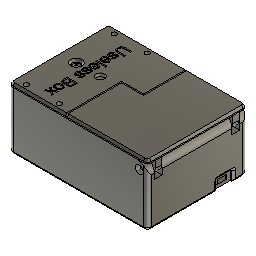
Smart_Useless_Box_box_v1 (Autodesk Fusion 360 design; units mm, degrees)
Autodesk Fusion 360 part; units mm, degrees
(part 1 of 2)
sketch "Base" plane through (0, 0, 0) normal (0, 0, 1) x (1, 0, 0) in component "Box Base"
  line L0 (50, -35) -> (-50, -35)
  line L1 (-50, -35) -> (-50, 35)
  line L2 (-50, 35) -> (50, 35)
  line L3 (50, 35) -> (50, -35)
  line L4 (50, -35) -> (-50, 35) construction
  line L5 (-50, -35) -> (50, 35) construction
  line L6 (50.5, -38.5) -> (-50.5, -38.5)
  line L7 (-53.5, -35.5) -> (-53.5, 35.5)
  line L8 (-50.5, 38.5) -> (50.5, 38.5)
  line L9 (53.5, 35.5) -> (53.5, -35.5)
  line L10 (53.5, -38.5) -> (-53.5, 38.5) construction
  line L11 (-53.5, -38.5) -> (53.5, 38.5) construction
  arc A0 (-53.5, -35.5) -> (-50.5, -38.5) centre (-50.5, -35.5) ccw
  arc A1 (-50.5, 38.5) -> (-53.5, 35.5) centre (-50.5, 35.5) ccw
  arc A2 (53.5, 35.5) -> (50.5, 38.5) centre (50.5, 35.5) ccw
  arc A3 (50.5, -38.5) -> (53.5, -35.5) centre (50.5, -35.5) ccw
  dimension "d5" = 100
  dimension "d6" = 70
  dimension "d7" = 77
  dimension "d8" = 107
  dimension "d9" = 3
  constraint perpendicular L0 L1
  constraint parallel L0 L2
  constraint parallel L1 L3
  constraint horizontal L0
  constraint coincident L4 origin
  constraint coincident L5 origin
  constraint perpendicular L6 L7
  constraint parallel L6 L8
  constraint parallel L7 L9
  constraint horizontal L6
  constraint coincident L10 origin
  constraint coincident L11 origin
  constraint coincident L11.start L6
  constraint coincident L11.start L7
  constraint tangent L6 A0
  constraint tangent L7 A0
  constraint coincident L10.end L7
  constraint coincident L10.end L8
  constraint tangent L7 A1
  constraint tangent L8 A1
  constraint equal A0 A1
  constraint coincident L11.end L8
  constraint coincident L11.end L9
  constraint tangent L8 A2
  constraint tangent L9 A2
  constraint equal A0 A2
  constraint coincident L10.start L9
  constraint coincident L10.start L6
  constraint tangent L9 A3
  constraint tangent L6 A3
  constraint equal A0 A3
  measures "d5" distance of L1.end L2.end
  measures "d6" distance of L0.end L1.end
  measures "d7" distance of L11.start L10.end
  measures "d8" distance of L10.end L11.end
  measures "d9" radius of A0
extrude "Extrude base bottom" add sketch "Base" along normal blind 2.4 contours L0 L1 L2 L3 makes body 1 in component "Box Base"
extrude "Extrude base wall" add sketch "Base" along normal blind 45 bodies 1 in component "Box Base"
chamfer "Chamfer bottom edges" distance 2 angle 35 8 edges at (-52.6213, -37.6213, 0) (-53.5, 0, 0) (-52.6213, 37.6213, 0) (0, 38.5, 0) (52.6213, 37.6213, 0) (53.5, 0, 0) (52.6213, -37.6213, 0) (0, -38.5, 0) measured on face at (-53.4154, -36.2073, 30) measured on face at (-16.8333, -12.8333, 0) measured on face at (-52.3545, 37.8582, 30) measured on face at (-16.8333, -12.8333, 0) measured on face at (51.8747, 38.1665, 30) measured on face at (-16.8333, -12.8333, 0) measured on face at (52, -38.0981, 30) measured on face at (-16.8333, -12.8333, 0) on bodies 1 in component "Box Base"
ref_plane "WorkPlane1" through (-10, 0, 23.7) normal (1, 0, 0) x (0, 1, 0) in component "Box Base"
sketch "Lid mount profile" plane through (-10, 0, 23.7) normal (1, 0, 0) x (0, 1, 0) in component "Box Base"
  line L0 (-35, -21.3) -> (-35, 21.3)
  line L1 (-35, 21.3) -> (35, 21.3)
  line L2 (35, -21.3) -> (35, 21.3)
  line L3 (-29.5, 21.3) -> (-35, 13.4452)
  line L4 (29.5, 21.3) -> (35, 13.4452)
  dimension "d28" = 5.5
  dimension "d29" = 35
  dimension "d30" = 7.8548
  dimension "d31" = 5.5
  dimension "d32" = 35
  constraint coincident L1 L3.start
  constraint coincident L0 L3.end
  constraint coincident L1 L4.start
  constraint coincident L2 L4.end
  measures "d28" distance of L0.end L3.start
  measures "d29" angle of L0 L3
  measures "d30" distance of L0.end L3.end
  measures "d31" distance of L1.end L4.start
  measures "d32" angle of L2 L4
extrude "Extrude lid mount profiles" add sketch "Lid mount profile" against normal up to surface (40 mm away) bodies 1 in component "Box Base"
sketch "Lid mount screws" plane through (0, 0, 45) normal (0, 0, 1) x (-1, 0, 0) in component "Box Base"
  line L0 (10, -35) -> (-50, -35)
  line L1 (-50, -35) -> (-50, 35)
  line L2 (-50, 35) -> (10, 35)
  line L3 (10, 35) -> (10, 29.5)
  line L4 (10, 29.5) -> (50, 29.5)
  line L5 (50, 29.5) -> (50, -29.5)
  line L6 (50, -29.5) -> (10, -29.5)
  line L7 (10, -29.5) -> (10, -35)
  arc A0 (53.5, 35.5) -> (50.5, 38.5) centre (50.5, 35.5) ccw
  line L8 (50.5, 38.5) -> (-50.5, 38.5)
  arc A1 (-50.5, 38.5) -> (-53.5, 35.5) centre (-50.5, 35.5) ccw
  line L9 (-53.5, 35.5) -> (-53.5, -35.5)
  arc A2 (-53.5, -35.5) -> (-50.5, -38.5) centre (-50.5, -35.5) ccw
  line L10 (-50.5, -38.5) -> (50.5, -38.5)
  arc A3 (50.5, -38.5) -> (53.5, -35.5) centre (50.5, -35.5) ccw
  line L11 (53.5, -35.5) -> (53.5, 35.5)
  line L12 (44.5, -29.5) -> (44.5, -38.5) construction
  line L13 (44.5, -34) -> (19, -34) construction
  line L14 (53.5, 0) -> (-53.5, 0) construction
  circle A4 centre (44.5, -34) radius 1.5
  circle A5 centre (19, -34) radius 1.5
  circle A6 centre (19, 34) radius 1.5
  circle A7 centre (44.5, 34) radius 1.5
  dimension "d36" = 9
  dimension "d37" = 9
  dimension "d38" = 3
  dimension "d39" = 3
  constraint coincident L6 L12.start
  constraint coincident L10 L12.end
  constraint perpendicular L10 L12
  constraint midpoint L12 L13.start
  constraint perpendicular L12 L13
  constraint midpoint L11 L14.start
  constraint midpoint L9 L14.end
  constraint coincident L13.start A4.centre
  constraint coincident L13.end A5.centre
  constraint symmetric L14 A4 A7
  constraint symmetric L14 A5 A6
  measures "d36" distance of L11 L12
  measures "d37" distance of L7 L13.end
  measures "d38" diameter of A4
  measures "d39" diameter of A5
extrude "Extrude5" cut sketch "Lid mount screws" against normal blind 15 contours A4 | A5 | A6 | A7 bodies 1 in component "Box Base"
chamfer "Chamfer screw hole edges" distance 1 angle 45 4 edges at (-43.1015, 33.4576, 45) (-17.6015, 33.4576, 45) (-43.1015, -34.5424, 45) (-17.6015, -34.5424, 45) on bodies 1 in component "Box Base"
sketch "Board support" plane through (0, 0, 2.4) normal (0, 0, 1) x (-1, 0, 0) in component "Box Base"
  line L0 (-50, -35) -> (50, -35)
  line L1 (50, -35) -> (50, 35)
  line L2 (50, 35) -> (-50, 35)
  line L3 (-50, 35) -> (-50, -35)
  line L4 (-50, -35) -> (-15, -35)
  line L5 (-15, -35) -> (-15, -8.5)
  line L6 (-15, -8.5) -> (-50, -8.5)
  line L7 (-50, -8.5) -> (-50, -35)
  line L8 (-15, -35) -> (-13, -35)
  line L9 (-13, -6.5) -> (-50, -6.5)
  line L10 (-50, -8.5) -> (-50, -6.5)
  line L11 (-13, -6.5) -> (-13, -35)
  line L12 (-19, -35) -> (-19, -8.5)
  dimension "d50" = 35
  dimension "d51" = 26.5
  dimension "d52" = 2
  dimension "d53" = 2
  dimension "d56" = 4
  constraint horizontal L4
  constraint vertical L5
  constraint horizontal L6
  constraint vertical L7
  constraint coincident L0.start L3.end
  constraint coincident L0 L8.end
  constraint perpendicular L5 L8
  constraint coincident L3 L9.end
  constraint perpendicular L3 L9
  constraint perpendicular L8 L11
  constraint coincident L4 L12.start
  constraint coincident L6 L12.end
  constraint perpendicular L6 L12
  measures "d50" distance of L0.start L4.end
  measures "d51" distance of L0.start L6.end
  measures "d52" distance of L4.end L8.end
  measures "d53" distance of L6 L9
  measures "d56" distance of L5 L12
extrude "Extrude board base support" add sketch "Board support" along normal blind 2 contours L0 L4 L5 L6 L12 bodies 1 in component "Box Base"
extrude "Extrude board wall support" add sketch "Board support" along normal blind 7 contours L0 L3 L5 L6 L8 L9 L10 L11 bodies 1 in component "Box Base"
sketch "USB hole" plane through (53.5, 0, 0) normal (1, 0, 0) x (0, 1, 0) in component "Box Base"
  line L0 (-35.5, 2) -> (35.5, 2)
  line L1 (35.5, 2) -> (35.5, 45)
  line L2 (35.5, 45) -> (-35.5, 45)
  line L3 (-35.5, 45) -> (-35.5, 2)
  line L4 (8.5, 2.4) -> (35, 2.4)
  line L5 (25.5, 2.4) -> (18, 2.4)
  line L6 (18, 2.4) -> (18, 5.6)
  line L7 (18, 5.6) -> (25.5, 5.6)
  line L8 (25.5, 5.6) -> (25.5, 2.4)
  line L9 (25.5, 2.4) -> (18, 5.6) construction
  line L10 (18, 2.4) -> (25.5, 5.6) construction
  line L11 (28, -0.1) -> (15.5, -0.1)
  line L12 (15.5, -0.1) -> (15.5, 7.1)
  line L13 (16.5, 8.1) -> (27, 8.1)
  line L14 (28, 7.1) -> (28, -0.1)
  line L15 (28, -0.1) -> (15.5, 8.1) construction
  line L16 (15.5, -0.1) -> (28, 8.1) construction
  arc A0 (16.5, 8.1) -> (15.5, 7.1) centre (16.5, 7.1) ccw
  arc A1 (28, 7.1) -> (27, 8.1) centre (27, 7.1) ccw
  point P0 (21.75, 4)
  point P1 (21.75, 4)
  dimension "d69" = 7.5
  dimension "d70" = 3.2
  dimension "d71" = 12.5
  dimension "d72" = 8.2
  dimension "d73" = 1
  constraint perpendicular L5 L6
  constraint parallel L5 L7
  constraint parallel L6 L8
  constraint horizontal L5
  constraint coincident L9 P1
  constraint coincident L10 P1
  constraint midpoint L4 L5
  constraint perpendicular L11 L12
  constraint parallel L11 L13
  constraint parallel L12 L14
  constraint horizontal L11
  constraint coincident L15 P1
  constraint coincident L16 P1
  constraint coincident P1 P0
  constraint coincident L15.end L12
  constraint coincident L15.end L13
  constraint tangent L12 A0
  constraint tangent L13 A0
  constraint coincident L16.end L13
  constraint coincident L16.end L14
  constraint tangent L13 A1
  constraint tangent L14 A1
  constraint equal A0 A1
  measures "d69" distance of L6.end L7.end
  measures "d70" distance of L5.end L6.end
  measures "d71" distance of L15.end L16.end
  measures "d72" distance of L11.end L15.end
  measures "d73" radius of A0
extrude "Cut USB hole" cut sketch "USB hole" against normal up to surface (3.5 mm away) contours L4 L5 L6 L7 L8 bodies 1 in component "Box Base"
extrude "Cut USB cable hole" cut sketch "USB hole" against normal blind 2.5 contours L0 L4 L5 L12 L14 | L0 L11 L12 L14 | L4 L6 L7 L8 L12 L13 L14 A0 A1 bodies 1 in component "Box Base"
chamfer "Chamfer USB edges" distance 2 angle 35 5 edges at (53.5, 15.5, 4.55) (53.5, 15.7929, 7.8071) (53.5, 21.75, 8.1) (53.5, 27.7071, 7.8071) (53.5, 28, 4.55) measured on face at (53.5, 5.3487, 32.6637) measured on face at (53.5, 5.3487, 32.6637) measured on face at (53.5, 5.3487, 32.6637) measured on face at (53.5, 5.3487, 32.6637) measured on face at (53.5, 5.3487, 32.6637) on bodies 1 in component "Box Base"
sketch "Shaft" plane through (0, -38.5, 0) normal (0, -1, 0) x (1, 0, 0) in component "Box Base"
  line L0 (-50.5, 2) -> (50.5, 2)
  line L1 (50.5, 2) -> (50.5, 45)
  line L2 (50.5, 45) -> (-50.5, 45)
  line L3 (-50.5, 45) -> (-50.5, 2)
  line L4 (53.5, 7.1) -> (53.5, 2)
  line L5 (53.5, 2) -> (53.5, 45)
  line L6 (53.5, 45) -> (53.5, 2)
  line L7 (53.5, 2) -> (53.5, 7.1)
  line L8 (53.5, 7.1) -> (53.5, 10.1)
  line L9 (53.5, 7.1) -> (53.5, 10.1)
  line L10 (-10, 45) -> (50, 45)
  line L11 (50, 2.4) -> (50, 45)
  circle A0 centre (47.3, 38.8) radius 1.5
  circle A1 centre (47.3, 38.8) radius 3.2
  circle A2 centre (47.3, 38.8) radius 6.2
  line L12 (41.1, 38.8) -> (41.1, 45)
  line L13 (42.2213, 35.2438) -> (50, 24.1346)
  spline S0 degree 5 poles (45.3, 45) (45.5877, 44.9597) (46.1522, 44.8682) (46.9666, 44.6986) (47.9866, 44.4066) (49.1443, 43.9243) (50.1744, 43.3144) (51.0663, 42.5663) (51.8144, 41.6744) (52.4243, 40.6443) (52.9066, 39.4866) (53.1986, 38.4666) (53.3682, 37.6522) (53.4597, 37.0877) (53.5, 36.8) knots 0 0 0 0 0 0 0.1 0.2 0.3 0.4 0.5 0.6 0.7 0.8 0.9 1 1 1 1 1 1
  line L14 (47.3, 38.8) -> (53.5, 45) construction
  line L15 (53.5, 45) -> (50, 45)
  point P0 (51.0304, 42.5304)
  dimension "d99" = 3
  dimension "d100" = 6.4
  dimension "d101" = 12.4
  dimension "d103" = 6.2
  dimension "d104" = 6.2
  dimension "d105" = 35
  dimension "d123" = 8.2
  dimension "d124" = 8.2
  constraint concentric A0 A1
  constraint concentric A0 A2
  constraint coincident A2 L12.start
  constraint tangent A2 L12
  constraint coincident L10 L12.end
  constraint perpendicular L2 L12
  constraint coincident A2 L13.start
  constraint tangent A2 L13
  constraint coincident L11 L13.end
  constraint coincident L10 S0.start
  constraint coincident L5 S0.end
  constraint coincident A0.centre A1.centre
  constraint coincident L5.end L6.start
  constraint coincident P0 L14
  constraint coincident L10.end L11.end
  measures "d99" diameter of A0
  measures "d100" diameter of A1
  measures "d101" diameter of A2
  measures "d103" distance of L2 A0.centre
  measures "d104" distance of L6 A0.centre
  measures "d105" angle of L11 L13
  measures "d123" distance of S0.start L5.end
  measures "d124" distance of S0.end L5.end
extrude "Extrude20" cut sketch "Shaft" against normal up to surface (77 mm away) contours L1 A2 S0 | L5 L6 A2 S0 | L1 L11 A2 S0 | L1 L5 L6 A2 L15 | L2 L10 A2 S0 | L1 L2 L11 A2 L15 | L11 A2 S0 | L2 L10 L11 A2 picked at (52.3629, 41.2358) bodies 1 in component "Box Base"
extrude "Extrude shaft case" add sketch "Shaft" against normal up to surface (73.5 mm away) contours L11 A1 A2 S0 | L11 A2 L13 | L2 L10 A2 L12 S0 | L11 A1 | L2 L10 A2 S0 | L11 A2 S0 | L2 L10 L11 A2 | A0 picked at (49.6, 38.8) bodies 1 in component "Box Base"
extrude "Cut shaft screw hole" cut sketch "Shaft" against normal up to surface (77 mm away) contours A0 bodies 1 in component "Box Base"
extrude "Cut shaft screw head hole front" cut sketch "Shaft" against normal blind 3.5 contours L11 A1 | L11 A1 bodies 1 in component "Box Base"
sketch "Shaft head hole back" plane through (0, 38.5, 0) normal (0, 1, 0) x (-1, 0, 0) in component "Box Base"
  circle A0 centre (-47.3, 38.8) radius 1.5
  line L0 (-50.5, 2) -> (50.5, 2)
  line L1 (50.5, 2) -> (50.5, 45)
  line L2 (50.5, 45) -> (-45.3, 45)
  line L3 (-50.5, 43.0074) -> (-50.5, 2)
  circle A1 centre (-47.3, 38.8) radius 3.2
  spline S0 degree 5 poles (-45.3, 45) (-45.5877, 44.9597) (-46.1522, 44.8682) (-46.9666, 44.6986) (-47.9866, 44.4066) (-49.0021, 43.9836) (-49.7129, 43.5838) (-50.175, 43.2634) (-50.43, 43.0639) (-50.5, 43.0074) knots 0 0 0 0 0 0 0.1 0.2 0.3 0.4 0.438574 0.438574 0.438574 0.438574 0.438574 0.438574
extrude "Cut shaft screw head hole back" cut sketch "Shaft head hole back" against normal blind 3.5 contours A1 bodies 1 in component "Box Base"
sketch "Shaft top mount holes" plane through (0, 0, 45) normal (0, 0, 1) x (-1, 0, 0) in component "Box Base"
  line L0 (50.5, 38.5) -> (-50, 38.5)
  line L1 (-45.3, -38.5) -> (50.5, -38.5)
  arc A0 (50.5, -38.5) -> (53.5, -35.5) centre (50.5, -35.5) ccw
  line L2 (53.5, -35.5) -> (53.5, 35.5)
  arc A1 (53.5, 35.5) -> (50.5, 38.5) centre (50.5, 35.5) ccw
  line L3 (-41.1, 35) -> (10, 35)
  line L4 (10, 35) -> (10, 29.5)
  line L5 (10, 29.5) -> (50, 29.5)
  line L6 (50, 29.5) -> (50, -29.5)
  line L7 (50, -29.5) -> (10, -29.5)
  line L8 (10, -29.5) -> (10, -35)
  line L9 (10, -35) -> (-41.1, -35)
  line L10 (-41.1, -35) -> (-41.1, 35)
  circle A2 centre (44.5, 34) radius 2.5
  circle A3 centre (44.5, -34) radius 2.5
  circle A4 centre (19, -34) radius 2.5
  circle A5 centre (19, 34) radius 2.5
  line L11 (-41.1, -33) -> (-53.5, -33)
  line L12 (-53.5, -33) -> (-53.5, -27)
  line L13 (-53.5, -27) -> (-41.1, -27)
  line L14 (-41.1, -27) -> (-41.1, -33)
  line L15 (-45.3, -35) -> (-45.3, -38.5)
  line L16 (-50, 38.5) -> (-50, -35)
  line L17 (-50, -35) -> (-45.3, -35)
  line L18 (53.5, 0) -> (-50, 0) construction
  line L19 (-41.1, 33) -> (-53.5, 33)
  line L20 (-53.5, 33) -> (-53.5, 27)
  line L21 (-53.5, 27) -> (-41.1, 27)
  line L22 (-41.1, 27) -> (-41.1, 33)
  dimension "d115" = 6
  dimension "d130" = 2
  constraint horizontal L11
  constraint vertical L12
  constraint horizontal L13
  constraint vertical L14
  constraint midpoint L2 L18.start
  constraint coincident L16 L18.end
  constraint perpendicular L16 L18
  constraint symmetric L11.start L18 L19.start
  constraint symmetric L11.end L18 L19.end
  constraint symmetric L12.end L18 L20.end
  constraint symmetric L13.end L18 L21.end
  measures "d115" distance of L11 L13
  measures "d130" distance of L11 L15.start
extrude "Cut shaft top mount holes" cut sketch "Shaft top mount holes" against normal blind 12.4 contours L10 L16 L19 L21 L22 | L16 L19 L20 L21 | L11 L12 L13 L16 | L10 L11 L13 L14 L16 bodies 1 in component "Box Base"
extrude "Cut shaft roundover" cut sketch "Shaft" against normal up to surface (77 mm away) contours L1 A2 S0 | L5 L6 A2 S0 | L1 L11 A2 S0 | L1 L5 L6 A2 L15 | L2 L10 A2 S0 | L1 L2 L11 A2 L15 | L11 A2 S0 | L2 L10 L11 A2 picked at (52.3629, 41.2358) bodies 1 in component "Box Base"
sketch "Top" plane through (0, 0, 45) normal (0, 0, 1) x (-1, 0, 0) in component "Fixed Lid"
  circle A0 centre (44.5, 34) radius 2.5
  circle A1 centre (44.5, -34) radius 2.5
  circle A2 centre (19, -34) radius 2.5
  circle A3 centre (19, 34) radius 2.5
  line L0 (-45.3, 38.5) -> (-45.3, 33)
  line L1 (-45.3, 33) -> (-41.1, 33)
  line L2 (-41.1, 33) -> (-41.1, 35)
  line L3 (-41.1, 35) -> (10, 35)
  line L4 (10, 35) -> (10, 29.5)
  line L5 (10, 29.5) -> (50, 29.5)
  line L6 (50, 29.5) -> (50, -29.5)
  line L7 (50, -29.5) -> (10, -29.5)
  line L8 (10, -29.5) -> (10, -35)
  line L9 (10, -35) -> (-41.1, -35)
  line L10 (-41.1, -35) -> (-41.1, -33)
  line L11 (-41.1, -33) -> (-45.3, -33)
  line L12 (-45.3, -33) -> (-45.3, -38.5)
  line L13 (-45.3, -38.5) -> (50.5, -38.5)
  arc A4 (50.5, -38.5) -> (53.5, -35.5) centre (50.5, -35.5) ccw
  line L14 (53.5, -35.5) -> (53.5, 35.5)
  arc A5 (53.5, 35.5) -> (50.5, 38.5) centre (50.5, 35.5) ccw
  line L15 (50.5, 38.5) -> (-45.3, 38.5)
  line L16 (10, -38.5) -> (10, 38.5)
  circle A6 centre (19, -34) radius 1.9
  circle A7 centre (44.5, -34) radius 1.9
  circle A8 centre (44.5, 34) radius 1.9
  circle A9 centre (19, 34) radius 1.9
  line L17 (0, 0) -> (53.5, 0) construction
  circle A10 centre (21.5, 0) radius 3.35
  line L18 (-7, -38.5) -> (-7, -5)
  line L19 (-7, -5) -> (10, -5)
  circle A11 centre (40, 0) radius 3.1
  line L20 (48, -5) -> (32, -5)
  line L21 (32, -5) -> (32, 16)
  line L22 (32, 16) -> (48, 16)
  line L23 (48, 16) -> (48, -5)
  line L24 (50, 18) -> (50, -7)
  line L25 (50, -7) -> (30, -7)
  line L26 (30, -7) -> (30, 18)
  line L27 (30, 18) -> (50, 18)
  line L28 (50, -29.5) -> (50, 29.5) construction
  line L29 (40, -5) -> (40, 16) construction
  dimension "d132" = 3.8
  dimension "d133" = 3.8
  dimension "d134" = 3.8
  dimension "d135" = 3.8
  dimension "d138" = 6.7
  dimension "d140" = 11.5
  dimension "d143" = 17
  dimension "d145" = 5
  dimension "d152" = 6.2
  dimension "d156" = 16
  dimension "d157" = 21
  dimension "d160" = 5
  constraint coincident L13 L16.start
  constraint coincident L15 L16.end
  constraint perpendicular L15 L16
  constraint collinear L8 L16
  constraint concentric A2 A6
  constraint concentric A1 A7
  constraint concentric A0 A8
  constraint concentric A3 A9
  constraint coincident L17.start origin
  constraint midpoint L14 L17.end
  constraint coincident L17 A10.centre
  constraint coincident L13 L18.start
  constraint perpendicular L13 L18
  constraint coincident L16 L19.end
  constraint perpendicular L16 L19
  constraint coincident L17 A11.centre
  constraint horizontal L20
  constraint vertical L21
  constraint horizontal L22
  constraint vertical L23
  constraint coincident L6.end L7.start
  constraint coincident L5.end L6.start
  constraint coincident L24 L5.end
  constraint midpoint L20 L29.start
  constraint midpoint L22 L29.end
  constraint coincident A11.centre L29
  measures "d132" diameter of A6
  measures "d133" diameter of A7
  measures "d134" diameter of A8
  measures "d135" diameter of A9
  measures "d138" diameter of A10
  measures "d140" distance of L16 A10.centre
  measures "d143" distance of L16 L18
  measures "d145" distance of L17.start L19
  measures "d152" diameter of A11
  measures "d156" distance of L20.start L20.end
  measures "d157" distance of L20.start L22.end
  measures "d160" distance of A11.centre L20
extrude "Extrude fixed lid" add sketch "Top" along normal blind 2.6 separate body contours A0 | A1 | A2 | A3 | L4 L5 L6 L7 L8 L13 A4 L14 A5 L15 L16 L24 | L5 L6 L7 L16 L25 L26 L27 | L8 L9 L16 L18 L19 | L6 L24 L25 L26 L27 | L9 L13 L16 L18 | L20 L21 L22 L23 makes body 2 in component "Fixed Lid"
chamfer "Chamfer1" distance 1.2 angle 55 6 edges at (-21.75, 38.5, 47.6) (-52.6213, 37.6213, 47.6) (-53.5, 0, 47.6) (-52.6213, -37.6213, 47.6) (-30.25, -38.5, 47.6) (-37.1098, -1.121, 47.6) measured on face at (-6.8691, 24.2359, 47.6) measured on face at (-6.8691, 24.2359, 47.6) measured on face at (-6.8691, 24.2359, 47.6) measured on face at (-6.8691, 24.2359, 47.6) measured on face at (-6.8691, 24.2359, 47.6) measured on face at (-6.8691, 24.2359, 47.6) on bodies 2 in component "Fixed Lid"
sketch "Bottom" plane through (0, 0, 45) normal (0, 0, -1) x (1, 0, 0) in component "Fixed Lid"
  circle A0 centre (-21.5, 0) radius 3.35
  circle A1 centre (-40, 0) radius 3.1
  circle A2 centre (-19, 34) radius 1.9
  circle A3 centre (-44.5, 34) radius 1.9
  circle A4 centre (-44.5, -34) radius 1.9
  circle A5 centre (-19, -34) radius 1.9
  line L0 (-50.5, -38.5) -> (7, -38.5)
  line L1 (7, -38.5) -> (7, -5)
  line L2 (7, -5) -> (-10, -5)
  line L3 (-10, -5) -> (-10, 38.5)
  line L4 (-10, 38.5) -> (-50.5, 38.5)
  arc A6 (-50.5, 38.5) -> (-53.5, 35.5) centre (-50.5, 35.5) ccw
  line L5 (-53.5, 35.5) -> (-53.5, -35.5)
  arc A7 (-53.5, -35.5) -> (-50.5, -38.5) centre (-50.5, -35.5) ccw
  line L6 (-50, -7) -> (-30, -7)
  line L7 (-30, -7) -> (-30, 18)
  line L8 (-50, 18) -> (-50, -7)
  line L9 (-30, 18) -> (-50, 18)
  line L10 (-48, -5) -> (-32, -5)
  line L11 (-32, -5) -> (-32, 16)
  line L12 (-48, 16) -> (-48, -5)
  line L13 (-32, 16) -> (-48, 16)
  line L14 (7, -38.5) -> (7, -5)
  line L15 (7, -23.5) -> (1.6, -23.5)
  line L16 (1.6, -23.5) -> (1.6, -15)
  line L17 (1.6, -15) -> (7, -15)
  line L18 (7, -15) -> (7, -23.5)
  line L19 (-21.6, -23.5) -> (-27, -23.5)
  line L20 (-27, -23.5) -> (-27, -15)
  line L21 (-27, -15) -> (-21.6, -15)
  line L22 (-21.6, -15) -> (-21.6, -23.5)
  line L23 (-42.6, -5) -> (-48, -5)
  line L24 (-48, -5) -> (-48, 0.4)
  line L25 (-48, 0.4) -> (-42.6, 0.4)
  line L26 (-42.6, 0.4) -> (-42.6, -5)
  line L27 (-42.6, -5) -> (-48, 0.4) construction
  line L28 (-48, -5) -> (-42.6, 0.4) construction
  line L29 (-32, -5) -> (-37.4, -5)
  line L30 (-37.4, -5) -> (-37.4, 0.4)
  line L31 (-37.4, 0.4) -> (-32, 0.4)
  line L32 (-32, 0.4) -> (-32, -5)
  line L33 (-32, -5) -> (-37.4, 0.4) construction
  line L34 (-37.4, -5) -> (-32, 0.4) construction
  circle A8 centre (-45.3, -2.3) radius 1.25
  circle A9 centre (-34.7, -2.3) radius 1.25
  arc A10 (-42.6, -2.3) -> (-45.3, 0.4) centre (-45.3, -2.3) ccw
  arc A11 (-34.7, 0.4) -> (-37.4, -2.3) centre (-34.7, -2.3) ccw
  point P0 (-45.3, -2.3)
  point P1 (-34.7, -2.3)
  dimension "d170" = 15
  dimension "d171" = 8.5
  dimension "d172" = 5.4
  dimension "d173" = 15
  dimension "d174" = 8.5
  dimension "d175" = 5.4
  dimension "d176" = 23.2
  dimension "d192" = 5.4
  dimension "d193" = 5.4
  dimension "d194" = 5.4
  dimension "d195" = 5.4
  dimension "d196" = 2.5
  dimension "d197" = 2.5
  constraint horizontal L15
  constraint vertical L16
  constraint horizontal L17
  constraint vertical L18
  constraint coincident L14 L15.start
  constraint horizontal L19
  constraint vertical L20
  constraint horizontal L21
  constraint vertical L22
  constraint perpendicular L23 L24
  constraint parallel L23 L25
  constraint parallel L24 L26
  constraint horizontal L23
  constraint coincident L27 P0
  constraint coincident L28 P0
  constraint coincident L10.start L12.end
  constraint perpendicular L29 L30
  constraint parallel L29 L31
  constraint parallel L30 L32
  constraint horizontal L29
  constraint coincident L33 P1
  constraint coincident L34 P1
  constraint coincident L10.end L11.start
  constraint coincident P0 A8.centre
  constraint coincident P1 A9.centre
  constraint midpoint L26 A10.start
  constraint midpoint L25 A10.end
  constraint midpoint L30 A11.end
  constraint midpoint L31 A11.start
  measures "d170" distance of origin L17
  measures "d171" distance of L15.end L16.end
  measures "d172" distance of L15.start L15.end
  measures "d173" distance of origin L21
  measures "d174" distance of L19.end L20.end
  measures "d175" distance of L19.start L19.end
  measures "d176" distance of L16 L22
  measures "d192" distance of L24.end L25.end
  measures "d193" distance of L10.start L24.end
  measures "d194" distance of L30.end L31.end
  measures "d195" distance of L29.end L30.end
  measures "d196" diameter of A8
  measures "d197" diameter of A9
extrude "Extrude6" add sketch "Bottom" along normal blind 1.6 contours A1 L10 L11 L29 L30 L31 L32 A11 | A1 A11 | A1 A10 | A1 L10 L12 L23 L24 L25 L26 A10 bodies 2 in component "Fixed Lid"
extrude "Extrude motor mounts" add sketch "Bottom" along normal blind 13 contours L1 L14 L15 L16 L17 L18 | L19 L20 L21 L22 bodies 2 in component "Fixed Lid"
extrude "Extrude sensor wall support" add sketch "Bottom" along normal blind 4 contours L6 L7 L8 L9 bodies 2 in component "Fixed Lid"
sketch "Motor mounts" plane through (0, 15, 0) normal (0, -1, 0) x (1, 0, 0) in component "Fixed Lid"
  line L0 (7, 45) -> (1.6, 45)
  line L1 (1.6, 45) -> (1.6, 32)
  line L2 (1.6, 32) -> (7, 32)
  line L3 (7, 32) -> (7, 45)
  line L4 (-21.6, 45) -> (-27, 45)
  line L5 (-27, 45) -> (-27, 32)
  line L6 (-27, 32) -> (-21.6, 32)
  line L7 (-21.6, 32) -> (-21.6, 45)
  line L8 (-24.3, 45) -> (-24.3, 32) construction
  line L9 (4.3, 45) -> (4.3, 32) construction
  circle A0 centre (-24.3, 38.7) radius 1.1
  circle A1 centre (4.3, 38.7) radius 1.1
  line L10 (-27, 45) -> (-21.6, 45)
  line L11 (1.6, 45) -> (7, 45)
  dimension "d179" = 2.2
  dimension "d180" = 2.2
  dimension "d182" = 6.3
  dimension "d183" = 6.3
  constraint midpoint L4 L8.start
  constraint midpoint L6 L8.end
  constraint midpoint L0 L9.start
  constraint midpoint L2 L9.end
  constraint coincident L8 A0.centre
  constraint coincident L9 A1.centre
  measures "d179" diameter of A0
  measures "d180" diameter of A1
  measures "d182" distance of A0.centre L10
  measures "d183" distance of A1.centre L11
extrude "Cut motor mount holes" cut sketch "Motor mounts" against normal up to surface (8.5 mm away) contours A0 | A1 bodies 2 in component "Fixed Lid"
fillet "Fillet1" radius 4 3 edges at (-27, 19.25, 45) (-24.3, 23.5, 45) (4.3, 23.5, 45) on bodies 2 in component "Fixed Lid"
sketch "Text" plane through (0, 0, 47.6) normal (0, 0, 1) x (-1, 0, 0) in component "Fixed Lid"
  circle A0 centre (21.5, 0) radius 3.35
  circle A1 centre (19, 34) radius 1.9
  circle A2 centre (44.5, 34) radius 1.9
  circle A3 centre (44.5, -34) radius 1.9
  circle A4 centre (19, -34) radius 1.9
  line L0 (-7, -37.3) -> (50.5, -37.3)
  arc A5 (50.5, -37.3) -> (52.3, -35.5) centre (50.5, -35.5) ccw
  line L1 (52.3, -35.5) -> (52.3, 35.5)
  arc A6 (52.3, 35.5) -> (50.5, 37.3) centre (50.5, 35.5) ccw
  line L2 (50.5, 37.3) -> (10, 37.3)
  line L3 (10, 37.3) -> (10, -5)
  line L4 (10, -5) -> (-7, -5)
  line L5 (-7, -5) -> (-7, -37.3)
  circle A7 centre (40, 0) radius 4.3
  line L6 (33.8228, -28.9087) -> (33.8228, 31.2798) construction
  line L7 (33.8228, 31.2798) -> (22.8228, 31.2798) construction
  line L8 (22.8228, 31.2798) -> (22.8228, -28.9087) construction
  line L9 (22.8228, -28.9087) -> (33.8228, -28.9087) construction
  text T0 "Useless Box" font "Arial" height 11 align ink ink in box 0 x 0 at (33.8228, -28.9087) x (0, 1) y (-1, 0) spacing 1 height is em
  constraint perpendicular L6 L7
  constraint parallel L6 L8
  constraint parallel L7 L9
extrude "Extrude5'" cut sketch "Text" against normal blind 1 text T0 bodies 2 in component "Fixed Lid"
sketch "Bottom (2)" plane through (0, 0, 45) normal (0, 0, 1) x (-1, 0, 0) in component "Moving Lid"
  circle A0 centre (44.5, 34) radius 2.5
  circle A1 centre (44.5, -34) radius 2.5
  circle A2 centre (19, -34) radius 2.5
  circle A3 centre (19, 34) radius 2.5
  line L0 (-45.3, 38.5) -> (-45.3, 33)
  line L1 (-45.3, 33) -> (-41.1, 33)
  line L2 (-41.1, 33) -> (-41.1, 35)
  line L3 (-41.1, 35) -> (10, 35)
  line L4 (10, 35) -> (10, 29.5)
  line L5 (10, 29.5) -> (50, 29.5)
  line L6 (50, 29.5) -> (50, -29.5)
  line L7 (50, -29.5) -> (10, -29.5)
  line L8 (10, -29.5) -> (10, -35)
  line L9 (10, -35) -> (-41.1, -35)
  line L10 (-41.1, -35) -> (-41.1, -33)
  line L11 (-41.1, -33) -> (-45.3, -33)
  line L12 (-45.3, -33) -> (-45.3, -38.5)
  line L13 (-45.3, -38.5) -> (50.5, -38.5)
  arc A4 (50.5, -38.5) -> (53.5, -35.5) centre (50.5, -35.5) ccw
  line L14 (53.5, -35.5) -> (53.5, 35.5)
  arc A5 (53.5, 35.5) -> (50.5, 38.5) centre (50.5, 35.5) ccw
  line L15 (50.5, 38.5) -> (-45.3, 38.5)
  circle A6 centre (40, 0) radius 4.3
  line L16 (-7, -37.3) -> (50.5, -37.3)
  arc A7 (50.5, -37.3) -> (52.3, -35.5) centre (50.5, -35.5) ccw
  line L17 (52.3, -35.5) -> (52.3, 35.5)
  arc A8 (52.3, 35.5) -> (50.5, 37.3) centre (50.5, 35.5) ccw
  line L18 (50.5, 37.3) -> (10, 37.3)
  line L19 (10, 37.3) -> (10, -5)
  line L20 (10, -5) -> (-7, -5)
  line L21 (-7, -5) -> (-7, -37.3)
  circle A9 centre (19, 34) radius 1.9
  circle A10 centre (44.5, -34) radius 1.9
  circle A11 centre (19, -34) radius 1.9
  circle A12 centre (21.5, 0) radius 3.35
  circle A13 centre (44.5, 34) radius 1.9
  spline S0 degree 3 poles (32.3472, -24.2366) (32.0988, -24.0953) (31.4834, -23.7453) (30.7695, -23.7469) (30.3438, -23.7478) knots 0 0 0 0 0.084501 0.209307 0.209307 0.209307 0.209307
  line L22 (30.3438, -23.7478) -> (25.7998, -23.7478)
  line L23 (25.7998, -23.7478) -> (25.7998, -22.7058)
  line L24 (25.7998, -22.7058) -> (30.3492, -22.7058)
  spline S1 degree 3 poles (30.3492, -22.7058) (30.7068, -22.7108) (31.3475, -22.7197) (31.9626, -22.8963) (32.2344, -22.9744) knots 0 0 0 0 0.106693 0.191173 0.191173 0.191173 0.191173
  spline S2 degree 3 poles (32.2344, -22.9744) (32.4581, -23.0849) (32.918, -23.3121) (33.2169, -23.7295) (33.3704, -23.9439) knots 0 0 0 0 0.073668 0.151407 0.151407 0.151407 0.151407
  spline S3 degree 3 poles (33.3704, -23.9439) (33.4978, -24.2095) (33.7761, -24.7895) (33.7969, -25.4341) (33.8081, -25.7835) knots 0 0 0 0 0.087434 0.190938 0.190938 0.190938 0.190938
  spline S4 degree 3 poles (33.8081, -25.7835) (33.7983, -26.1236) (33.7802, -26.7511) (33.5378, -27.3289) (33.4268, -27.5935) knots 0 0 0 0 0.101025 0.186391 0.186391 0.186391 0.186391
  spline S5 degree 3 poles (33.4268, -27.5935) (33.2862, -27.811) (33.0068, -28.2432) (32.55, -28.4802) (32.323, -28.5979) knots 0 0 0 0 0.076238 0.151547 0.151547 0.151547 0.151547
  spline S6 degree 3 poles (32.323, -28.5979) (32.0401, -28.6853) (31.3983, -28.8837) (30.7255, -28.8933) (30.3492, -28.8987) knots 0 0 0 0 0.088394 0.200567 0.200567 0.200567 0.200567
  line L25 (30.3492, -28.8987) -> (25.7998, -28.8987)
  line L26 (25.7998, -28.8987) -> (25.7998, -27.8567)
  line L27 (25.7998, -27.8567) -> (30.3438, -27.8567)
  spline S7 degree 3 poles (30.3438, -27.8567) (30.6429, -27.8556) (31.1555, -27.8538) (31.6498, -27.7213) (31.8558, -27.666) knots 0 0 0 0 0.08922 0.152949 0.152949 0.152949 0.152949
  spline S8 degree 3 poles (31.8558, -27.666) (32.0088, -27.5906) (32.3166, -27.4388) (32.5085, -27.154) (32.605, -27.0108) knots 0 0 0 0 0.050236 0.10109 0.10109 0.10109 0.10109
  spline S9 degree 3 poles (32.605, -27.0108) (32.6817, -26.8413) (32.8449, -26.4807) (32.8601, -26.0847) (32.8682, -25.8748) knots 0 0 0 0 0.055274 0.117592 0.117592 0.117592 0.117592
  spline S10 degree 3 poles (32.8682, -25.8748) (32.8605, -25.5342) (32.847, -24.9324) (32.4985, -24.4472) (32.3472, -24.2366) knots 0 0 0 0 0.099283 0.175461 0.175461 0.175461 0.175461
  spline S11 degree 3 poles (33.0079, -13.1936) (32.9979, -13.0252) (32.9786, -12.6994) (32.81, -12.4206) (32.7286, -12.2859) knots 0 0 0 0 0.049772 0.096252 0.096252 0.096252 0.096252
  spline S12 degree 3 poles (32.7286, -12.2859) (32.6139, -12.1645) (32.3629, -11.8985) (32.0221, -11.7632) (31.837, -11.6897) knots 0 0 0 0 0.049501 0.108413 0.108413 0.108413 0.108413
  line L28 (31.837, -11.6897) -> (31.9605, -10.6907)
  spline S13 degree 3 poles (31.9605, -10.6907) (32.2331, -10.7825) (32.7605, -10.9601) (33.1373, -11.3687) (33.3194, -11.5662) knots 0 0 0 0 0.084738 0.163983 0.163983 0.163983 0.163983
  spline S14 degree 3 poles (33.3194, -11.5662) (33.4602, -11.8026) (33.7593, -12.3046) (33.7877, -12.8896) (33.8028, -13.199) knots 0 0 0 0 0.081309 0.172615 0.172615 0.172615 0.172615
  spline S15 degree 3 poles (33.8028, -13.199) (33.777, -13.5883) (33.7276, -14.3328) (33.2567, -14.9088) (33.032, -15.1836) knots 0 0 0 0 0.113831 0.217681 0.217681 0.217681 0.217681
  spline S16 degree 3 poles (33.032, -15.1836) (32.7342, -15.3971) (32.0906, -15.8584) (31.2966, -15.8964) (30.8702, -15.9168) knots 0 0 0 0 0.107682 0.232636 0.232636 0.232636 0.232636
  spline S17 degree 3 poles (30.8702, -15.9168) (30.4295, -15.8967) (29.6116, -15.8593) (28.9438, -15.3914) (28.6358, -15.1755) knots 0 0 0 0 0.129168 0.239761 0.239761 0.239761 0.239761
  spline S18 degree 3 poles (28.6358, -15.1755) (28.404, -14.9057) (27.9291, -14.3528) (27.8707, -13.6251) (27.8409, -13.2527) knots 0 0 0 0 0.103932 0.212913 0.212913 0.212913 0.212913
  spline S19 degree 3 poles (27.8409, -13.2527) (27.8706, -12.8914) (27.9288, -12.1834) (28.3925, -11.6465) (28.6197, -11.3836) knots 0 0 0 0 0.105739 0.207218 0.207218 0.207218 0.207218
  spline S20 degree 3 poles (28.6197, -11.3836) (28.9217, -11.1724) (29.5769, -10.7143) (30.3788, -10.678) (30.8111, -10.6585) knots 0 0 0 0 0.10836 0.235079 0.235079 0.235079 0.235079
  spline S21 degree 3 poles (30.8111, -10.6585) (30.8469, -10.6588) (30.9328, -10.6596) (31.0188, -10.6623) (31.0689, -10.6638) knots 0 0 0 0 0.010743 0.025787 0.025787 0.025787 0.025787
  line L29 (31.0689, -10.6638) -> (31.0689, -14.9177)
  spline S22 degree 3 poles (31.0689, -14.9177) (31.3553, -14.8898) (31.8837, -14.8383) (32.3121, -14.5281) (32.5083, -14.386) knots 0 0 0 0 0.084508 0.155921 0.155921 0.155921 0.155921
  spline S23 degree 3 poles (32.5083, -14.386) (32.654, -14.2157) (32.9481, -13.872) (32.9878, -13.4211) (33.0079, -13.1936) knots 0 0 0 0 0.065486 0.132192 0.132192 0.132192 0.132192
  spline S24 degree 3 poles (33.0079, -4.6321) (32.9979, -4.4636) (32.9786, -4.1379) (32.81, -3.859) (32.7286, -3.7244) knots 0 0 0 0 0.049772 0.096251 0.096251 0.096251 0.096251
  spline S25 degree 3 poles (32.7286, -3.7244) (32.6139, -3.603) (32.3629, -3.337) (32.0221, -3.2017) (31.837, -3.1282) knots 0 0 0 0 0.049501 0.108413 0.108413 0.108413 0.108413
  line L30 (31.837, -3.1282) -> (31.9605, -2.1292)
  spline S26 degree 3 poles (31.9605, -2.1292) (32.2331, -2.2209) (32.7605, -2.3986) (33.1373, -2.8072) (33.3194, -3.0046) knots 0 0 0 0 0.084738 0.163983 0.163983 0.163983 0.163983
  spline S27 degree 3 poles (33.3194, -3.0046) (33.4602, -3.2411) (33.7593, -3.7431) (33.7877, -4.328) (33.8028, -4.6375) knots 0 0 0 0 0.081309 0.172615 0.172615 0.172615 0.172615
  spline S28 degree 3 poles (33.8028, -4.6375) (33.777, -5.0268) (33.7276, -5.7713) (33.2567, -6.3473) (33.032, -6.6221) knots 0 0 0 0 0.113832 0.217681 0.217681 0.217681 0.217681
  spline S29 degree 3 poles (33.032, -6.6221) (32.7342, -6.8356) (32.0906, -7.2969) (31.2966, -7.3349) (30.8702, -7.3552) knots 0 0 0 0 0.107682 0.232636 0.232636 0.232636 0.232636
  spline S30 degree 3 poles (30.8702, -7.3552) (30.4295, -7.3351) (29.6116, -7.2978) (28.9438, -6.8299) (28.6358, -6.614) knots 0 0 0 0 0.129168 0.239761 0.239761 0.239761 0.239761
  spline S31 degree 3 poles (28.6358, -6.614) (28.404, -6.3441) (27.9291, -5.7912) (27.8707, -5.0636) (27.8409, -4.6912) knots 0 0 0 0 0.103932 0.212913 0.212913 0.212913 0.212913
  spline S32 degree 3 poles (27.8409, -4.6912) (27.8706, -4.3299) (27.9288, -3.6219) (28.3925, -3.085) (28.6197, -2.822) knots 0 0 0 0 0.105739 0.207218 0.207218 0.207218 0.207218
  spline S33 degree 3 poles (28.6197, -2.822) (28.9217, -2.6109) (29.5769, -2.1528) (30.3788, -2.1165) (30.8111, -2.0969) knots 0 0 0 0 0.10836 0.235079 0.235079 0.235079 0.235079
  spline S34 degree 3 poles (30.8111, -2.0969) (30.8469, -2.0973) (30.9328, -2.0981) (31.0188, -2.1008) (31.0689, -2.1023) knots 0 0 0 0 0.010743 0.025787 0.025787 0.025787 0.025787
  line L31 (31.0689, -2.1023) -> (31.0689, -6.3562)
  spline S35 degree 3 poles (31.0689, -6.3562) (31.3553, -6.3283) (31.8837, -6.2767) (32.3121, -5.9665) (32.5083, -5.8245) knots 0 0 0 0 0.084508 0.155921 0.155921 0.155921 0.155921
  spline S36 degree 3 poles (32.5083, -5.8245) (32.654, -5.6542) (32.9481, -5.3105) (32.9878, -4.8596) (33.0079, -4.6321) knots 0 0 0 0 0.065486 0.132192 0.132192 0.132192 0.132192
  spline S37 degree 3 poles (33.8028, 1.1365) (33.7933, 0.8015) (33.7763, 0.1966) (33.4752, -0.3253) (33.3409, -0.5581) knots 0 0 0 0 0.098634 0.178087 0.178087 0.178087 0.178087
  spline S38 degree 3 poles (33.3409, -0.5581) (33.1603, -0.7361) (32.7764, -1.1144) (32.25, -1.2371) (31.9712, -1.302) knots 0 0 0 0 0.074607 0.158576 0.158576 0.158576 0.158576
  line L32 (31.9712, -1.302) -> (31.8208, -0.346)
  spline S39 degree 3 poles (31.8208, -0.346) (31.9981, -0.3107) (32.3348, -0.2437) (32.5838, -0.0087) (32.7017, 0.1025) knots 0 0 0 0 0.052996 0.100641 0.100641 0.100641 0.100641
  spline S40 degree 3 poles (32.7017, 0.1025) (32.7908, 0.2456) (32.9861, 0.5591) (33.0002, 0.9297) (33.0079, 1.1311) knots 0 0 0 0 0.049728 0.108971 0.108971 0.108971 0.108971
  spline S41 degree 3 poles (33.0079, 1.1311) (33.0033, 1.3298) (32.9951, 1.6837) (32.8154, 1.9866) (32.7366, 2.1194) knots 0 0 0 0 0.058403 0.104012 0.104012 0.104012 0.104012
  spline S42 degree 3 poles (32.7366, 2.1194) (32.645, 2.2133) (32.4689, 2.3938) (32.2197, 2.4261) (32.1001, 2.4416) knots 0 0 0 0 0.038117 0.073227 0.073227 0.073227 0.073227
  spline S43 degree 3 poles (32.1001, 2.4416) (31.9964, 2.4292) (31.7863, 2.4041) (31.6523, 2.24) (31.5845, 2.157) knots 0 0 0 0 0.030125 0.060991 0.060991 0.060991 0.060991
  spline S44 degree 3 poles (31.5845, 2.157) (31.5331, 2.0424) (31.3904, 1.7247) (31.309, 1.3856) (31.2569, 1.1687) knots 0 0 0 0 0.037608 0.104304 0.104304 0.104304 0.104304
  spline S45 degree 3 poles (31.2569, 1.1687) (31.1811, 0.8661) (31.0556, 0.3651) (30.867, -0.1154) (30.7923, -0.3057) knots 0 0 0 0 0.093451 0.15472 0.15472 0.15472 0.15472
  spline S46 degree 3 poles (30.7923, -0.3057) (30.7225, -0.4332) (30.5871, -0.6808) (30.3599, -0.8478) (30.2498, -0.9287) knots 0 0 0 0 0.043018 0.083508 0.083508 0.083508 0.083508
  spline S47 degree 3 poles (30.2498, -0.9287) (30.1307, -0.9906) (29.8907, -1.1154) (29.6206, -1.1323) (29.4844, -1.1409) knots 0 0 0 0 0.039778 0.080209 0.080209 0.080209 0.080209
  spline S48 degree 3 poles (29.4844, -1.1409) (29.3601, -1.1339) (29.1137, -1.12) (28.8893, -1.0172) (28.7781, -0.9663) knots 0 0 0 0 0.036983 0.073328 0.073328 0.073328 0.073328
  spline S49 degree 3 poles (28.7781, -0.9663) (28.6744, -0.9028) (28.4668, -0.7758) (28.3145, -0.586) (28.2383, -0.491) knots 0 0 0 0 0.036186 0.072411 0.072411 0.072411 0.072411
  spline S50 degree 3 poles (28.2383, -0.491) (28.1835, -0.4038) (28.0625, -0.2115) (27.9939, 0.0054) (27.9563, 0.124) knots 0 0 0 0 0.03077 0.0679 0.0679 0.0679 0.0679
  spline S51 degree 3 poles (27.9563, 0.124) (27.9227, 0.2578) (27.8537, 0.532) (27.8452, 0.8146) (27.8409, 0.9592) knots 0 0 0 0 0.041269 0.084536 0.084536 0.084536 0.084536
  spline S52 degree 3 poles (27.8409, 0.9592) (27.847, 1.171) (27.8587, 1.5729) (27.9779, 1.9567) (28.0342, 2.1382) knots 0 0 0 0 0.063228 0.119965 0.119965 0.119965 0.119965
  spline S53 degree 3 poles (28.0342, 2.1382) (28.0997, 2.2927) (28.2215, 2.5801) (28.4515, 2.7902) (28.5579, 2.8874) knots 0 0 0 0 0.049636 0.092371 0.092371 0.092371 0.092371
  spline S54 degree 3 poles (28.5579, 2.8874) (28.6838, 2.9627) (28.9578, 3.1266) (29.2717, 3.1875) (29.4414, 3.2204) knots 0 0 0 0 0.043668 0.095061 0.095061 0.095061 0.095061
  line L33 (29.4414, 3.2204) -> (29.5704, 2.2751)
  spline S55 degree 3 poles (29.5704, 2.2751) (29.4331, 2.2452) (29.1672, 2.1874) (28.9755, 1.9949) (28.8829, 1.9018) knots 0 0 0 0 0.04117 0.079724 0.079724 0.079724 0.079724
  spline S56 degree 3 poles (28.8829, 1.9018) (28.811, 1.7807) (28.652, 1.5128) (28.6415, 1.2002) (28.6358, 1.029) knots 0 0 0 0 0.041615 0.092013 0.092013 0.092013 0.092013
  spline S57 degree 3 poles (28.6358, 1.029) (28.6373, 0.8345) (28.64, 0.4993) (28.7922, 0.2028) (28.856, 0.0784) knots 0 0 0 0 0.057333 0.098767 0.098767 0.098767 0.098767
  spline S58 degree 3 poles (28.856, 0.0784) (28.9294, -0.0046) (29.0682, -0.1615) (29.2744, -0.1919) (29.3716, -0.2063) knots 0 0 0 0 0.032048 0.06061 0.06061 0.06061 0.06061
  spline S59 degree 3 poles (29.3716, -0.2063) (29.4328, -0.2013) (29.5558, -0.1912) (29.6585, -0.1226) (29.71, -0.0881) knots 0 0 0 0 0.018102 0.036374 0.036374 0.036374 0.036374
  spline S60 degree 3 poles (29.71, -0.0881) (29.7609, -0.04) (29.8723, 0.0653) (29.9342, 0.206) (29.9678, 0.2825) knots 0 0 0 0 0.020804 0.045551 0.045551 0.045551 0.045551
  spline S61 degree 3 poles (29.9678, 0.2825) (29.9978, 0.3777) (30.0869, 0.6604) (30.1638, 0.9466) (30.2149, 1.1365) knots 0 0 0 0 0.029943 0.088911 0.088911 0.088911 0.088911
  spline S62 degree 3 poles (30.2149, 1.1365) (30.2924, 1.4285) (30.4209, 1.9123) (30.5945, 2.3817) (30.6634, 2.5679) knots 0 0 0 0 0.090571 0.150073 0.150073 0.150073 0.150073
  spline S63 degree 3 poles (30.6634, 2.5679) (30.7268, 2.6948) (30.851, 2.9432) (31.0659, 3.1186) (31.1709, 3.2043) knots 0 0 0 0 0.042051 0.082236 0.082236 0.082236 0.082236
  spline S64 degree 3 poles (31.1709, 3.2043) (31.2926, 3.2716) (31.5496, 3.4138) (31.8434, 3.4279) (31.9981, 3.4353) knots 0 0 0 0 0.041152 0.086904 0.086904 0.086904 0.086904
  spline S65 degree 3 poles (31.9981, 3.4353) (32.1579, 3.4228) (32.4825, 3.3976) (32.7651, 3.2355) (32.9085, 3.1533) knots 0 0 0 0 0.047456 0.096374 0.096374 0.096374 0.096374
  spline S66 degree 3 poles (32.9085, 3.1533) (33.044, 3.0461) (33.3244, 2.8242) (33.4857, 2.5047) (33.5691, 2.3396) knots 0 0 0 0 0.051187 0.105937 0.105937 0.105937 0.105937
  spline S67 degree 3 poles (33.5691, 2.3396) (33.6372, 2.1526) (33.7788, 1.7642) (33.7946, 1.3509) (33.8028, 1.1365) knots 0 0 0 0 0.059313 0.123228 0.123228 0.123228 0.123228
  spline S68 degree 3 poles (33.5423, 17.4941) (33.5806, 17.3025) (33.6643, 16.8834) (33.6705, 16.4559) (33.6739, 16.2239) knots 0 0 0 0 0.05851 0.127942 0.127942 0.127942 0.127942
  line L34 (33.6739, 16.2239) -> (33.6739, 13.2214)
  line L35 (33.6739, 13.2214) -> (25.7998, 13.2214)
  line L36 (25.7998, 13.2214) -> (25.7998, 16.1755)
  spline S69 degree 3 poles (25.7998, 16.1755) (25.8048, 16.4492) (25.8139, 16.9441) (25.9693, 17.4133) (26.0389, 17.623) knots 0 0 0 0 0.081524 0.147454 0.147454 0.147454 0.147454
  spline S70 degree 3 poles (26.0389, 17.623) (26.1289, 17.7947) (26.3081, 18.1363) (26.6196, 18.3638) (26.7747, 18.477) knots 0 0 0 0 0.057303 0.114076 0.114076 0.114076 0.114076
  spline S71 degree 3 poles (26.7747, 18.477) (26.9403, 18.5671) (27.2651, 18.7437) (27.6335, 18.772) (27.814, 18.7859) knots 0 0 0 0 0.055853 0.109518 0.109518 0.109518 0.109518
  spline S72 degree 3 poles (27.814, 18.7859) (27.9805, 18.774) (28.3167, 18.7501) (28.6144, 18.5918) (28.7647, 18.512) knots 0 0 0 0 0.049487 0.099919 0.099919 0.099919 0.099919
  spline S73 degree 3 poles (28.7647, 18.512) (28.9079, 18.4053) (29.2075, 18.1821) (29.3895, 17.8553) (29.4844, 17.6848) knots 0 0 0 0 0.052956 0.110758 0.110758 0.110758 0.110758
  spline S74 degree 3 poles (29.4844, 17.6848) (29.5626, 17.9061) (29.7126, 18.3304) (30.0414, 18.6367) (30.1988, 18.7832) knots 0 0 0 0 0.06924 0.132763 0.132763 0.132763 0.132763
  spline S75 degree 3 poles (30.1988, 18.7832) (30.3771, 18.8952) (30.7416, 19.1242) (31.1715, 19.1527) (31.3912, 19.1672) knots 0 0 0 0 0.062133 0.127032 0.127032 0.127032 0.127032
  spline S76 degree 3 poles (31.3912, 19.1672) (31.5714, 19.1579) (31.9279, 19.1396) (32.257, 19.0017) (32.4197, 18.9336) knots 0 0 0 0 0.053694 0.106186 0.106186 0.106186 0.106186
  spline S77 degree 3 poles (32.4197, 18.9336) (32.5664, 18.8546) (32.8448, 18.7046) (33.054, 18.4681) (33.1529, 18.3562) knots 0 0 0 0 0.049539 0.093976 0.093976 0.093976 0.093976
  spline S78 degree 3 poles (33.1529, 18.3562) (33.2346, 18.23) (33.4078, 17.9625) (33.4958, 17.656) (33.5423, 17.4941) knots 0 0 0 0 0.044862 0.095055 0.095055 0.095055 0.095055
  spline S79 degree 3 poles (33.8028, 22.7927) (33.7752, 22.417) (33.7218, 21.6895) (33.2587, 21.128) (33.0347, 20.8564) knots 0 0 0 0 0.109984 0.212941 0.212941 0.212941 0.212941
  spline S80 degree 3 poles (33.0347, 20.8564) (32.733, 20.6414) (32.0741, 20.1719) (31.262, 20.1369) (30.8218, 20.1179) knots 0 0 0 0 0.108869 0.237762 0.237762 0.237762 0.237762
  spline S81 degree 3 poles (30.8218, 20.1179) (30.3417, 20.1399) (29.4586, 20.1805) (28.783, 20.7424) (28.4746, 20.9988) knots 0 0 0 0 0.13965 0.256857 0.256857 0.256857 0.256857
  spline S82 degree 3 poles (28.4746, 20.9988) (28.2898, 21.2615) (27.9112, 21.7995) (27.8647, 22.4565) (27.8409, 22.7927) knots 0 0 0 0 0.09447 0.1935 0.1935 0.1935 0.1935
  spline S83 degree 3 poles (27.8409, 22.7927) (27.8695, 23.1635) (27.9254, 23.8863) (28.3868, 24.444) (28.6116, 24.7156) knots 0 0 0 0 0.108608 0.211733 0.211733 0.211733 0.211733
  spline S84 degree 3 poles (28.6116, 24.7156) (28.9063, 24.9331) (29.537, 25.3986) (30.3226, 25.4401) (30.7412, 25.4621) knots 0 0 0 0 0.107511 0.230125 0.230125 0.230125 0.230125
  spline S85 degree 3 poles (30.7412, 25.4621) (31.0734, 25.4557) (31.671, 25.4441) (32.2266, 25.2279) (32.4734, 25.1318) knots 0 0 0 0 0.098704 0.177557 0.177557 0.177557 0.177557
  spline S86 degree 3 poles (32.4734, 25.1318) (32.6722, 25.0088) (33.0712, 24.762) (33.3259, 24.3681) (33.4537, 24.1704) knots 0 0 0 0 0.06919 0.13884 0.13884 0.13884 0.13884
  spline S87 degree 3 poles (33.4537, 24.1704) (33.5555, 23.9541) (33.761, 23.5176) (33.7888, 23.0358) (33.8028, 22.7927) knots 0 0 0 0 0.071002 0.143302 0.143302 0.143302 0.143302
  spline S88 degree 3 poles (33.8028, 6.6365) (33.7933, 6.3015) (33.7763, 5.6966) (33.4752, 5.1747) (33.3409, 4.9419) knots 0 0 0 0 0.098634 0.178087 0.178087 0.178087 0.178087
  spline S89 degree 3 poles (33.3409, 4.9419) (33.1603, 4.7639) (32.7764, 4.3856) (32.25, 4.2629) (31.9712, 4.198) knots 0 0 0 0 0.074607 0.158576 0.158576 0.158576 0.158576
  line L37 (31.9712, 4.198) -> (31.8208, 5.154)
  spline S90 degree 3 poles (31.8208, 5.154) (31.9981, 5.1893) (32.3348, 5.2563) (32.5838, 5.4913) (32.7017, 5.6025) knots 0 0 0 0 0.052996 0.100641 0.100641 0.100641 0.100641
  spline S91 degree 3 poles (32.7017, 5.6025) (32.7908, 5.7456) (32.9861, 6.0591) (33.0002, 6.4297) (33.0079, 6.6311) knots 0 0 0 0 0.049728 0.108971 0.108971 0.108971 0.108971
  spline S92 degree 3 poles (33.0079, 6.6311) (33.0033, 6.8298) (32.9951, 7.1837) (32.8154, 7.4866) (32.7366, 7.6194) knots 0 0 0 0 0.058403 0.104012 0.104012 0.104012 0.104012
  spline S93 degree 3 poles (32.7366, 7.6194) (32.645, 7.7133) (32.4689, 7.8938) (32.2197, 7.9261) (32.1001, 7.9416) knots 0 0 0 0 0.038117 0.073227 0.073227 0.073227 0.073227
  spline S94 degree 3 poles (32.1001, 7.9416) (31.9964, 7.9292) (31.7863, 7.9041) (31.6523, 7.74) (31.5845, 7.657) knots 0 0 0 0 0.030125 0.060991 0.060991 0.060991 0.060991
  spline S95 degree 3 poles (31.5845, 7.657) (31.5331, 7.5424) (31.3904, 7.2247) (31.309, 6.8856) (31.2569, 6.6687) knots 0 0 0 0 0.037608 0.104304 0.104304 0.104304 0.104304
  spline S96 degree 3 poles (31.2569, 6.6687) (31.1811, 6.3661) (31.0556, 5.8651) (30.867, 5.3846) (30.7923, 5.1943) knots 0 0 0 0 0.093451 0.15472 0.15472 0.15472 0.15472
  spline S97 degree 3 poles (30.7923, 5.1943) (30.7225, 5.0668) (30.5871, 4.8192) (30.3599, 4.6522) (30.2498, 4.5713) knots 0 0 0 0 0.043018 0.083508 0.083508 0.083508 0.083508
  spline S98 degree 3 poles (30.2498, 4.5713) (30.1307, 4.5094) (29.8907, 4.3846) (29.6206, 4.3677) (29.4844, 4.3591) knots 0 0 0 0 0.039778 0.080209 0.080209 0.080209 0.080209
  spline S99 degree 3 poles (29.4844, 4.3591) (29.3601, 4.3661) (29.1137, 4.38) (28.8893, 4.4828) (28.7781, 4.5337) knots 0 0 0 0 0.036983 0.073328 0.073328 0.073328 0.073328
  spline S100 degree 3 poles (28.7781, 4.5337) (28.6744, 4.5972) (28.4668, 4.7242) (28.3145, 4.914) (28.2383, 5.009) knots 0 0 0 0 0.036186 0.072411 0.072411 0.072411 0.072411
  spline S101 degree 3 poles (28.2383, 5.009) (28.1835, 5.0962) (28.0625, 5.2885) (27.9939, 5.5054) (27.9563, 5.624) knots 0 0 0 0 0.03077 0.0679 0.0679 0.0679 0.0679
  spline S102 degree 3 poles (27.9563, 5.624) (27.9227, 5.7578) (27.8537, 6.032) (27.8452, 6.3146) (27.8409, 6.4592) knots 0 0 0 0 0.041269 0.084536 0.084536 0.084536 0.084536
  spline S103 degree 3 poles (27.8409, 6.4592) (27.847, 6.671) (27.8587, 7.0729) (27.9779, 7.4567) (28.0342, 7.6382) knots 0 0 0 0 0.063228 0.119965 0.119965 0.119965 0.119965
  spline S104 degree 3 poles (28.0342, 7.6382) (28.0997, 7.7927) (28.2215, 8.0801) (28.4515, 8.2902) (28.5579, 8.3874) knots 0 0 0 0 0.049636 0.092371 0.092371 0.092371 0.092371
  spline S105 degree 3 poles (28.5579, 8.3874) (28.6838, 8.4627) (28.9578, 8.6266) (29.2717, 8.6875) (29.4414, 8.7204) knots 0 0 0 0 0.043668 0.095061 0.095061 0.095061 0.095061
  line L38 (29.4414, 8.7204) -> (29.5704, 7.7751)
  spline S106 degree 3 poles (29.5704, 7.7751) (29.4331, 7.7452) (29.1672, 7.6874) (28.9755, 7.4949) (28.8829, 7.4018) knots 0 0 0 0 0.04117 0.079724 0.079724 0.079724 0.079724
  spline S107 degree 3 poles (28.8829, 7.4018) (28.811, 7.2807) (28.652, 7.0128) (28.6415, 6.7002) (28.6358, 6.529) knots 0 0 0 0 0.041615 0.092013 0.092013 0.092013 0.092013
  spline S108 degree 3 poles (28.6358, 6.529) (28.6373, 6.3345) (28.64, 5.9993) (28.7922, 5.7028) (28.856, 5.5784) knots 0 0 0 0 0.057333 0.098767 0.098767 0.098767 0.098767
  spline S109 degree 3 poles (28.856, 5.5784) (28.9294, 5.4954) (29.0682, 5.3385) (29.2744, 5.3081) (29.3716, 5.2937) knots 0 0 0 0 0.032049 0.060611 0.060611 0.060611 0.060611